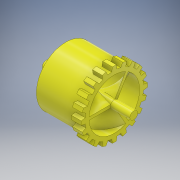
# Autodesk Inventor part: Rotator
Saved by Autodesk Inventor 2018.3 (Build 223284000, 284)
## iProperties
Created: 2020-03-27
Part Number: Rotator
Material: Generic
Document SubType Name: Modeling
Designer: ToreDenStore
Density: 1 g/cm^3
Appearance: Default
Author: ToreDenStore
Autodesk Inventor part; units mm, degrees
ref_plane "YZ Plane" through (0, 0, 0) normal (1, 0, 0) x (0, 1, 0)
ref_plane "XZ Plane" through (0, 0, 0) normal (0, 1, 0) x (-1, 0, 0)
ref_plane "XY Plane" through (0, 0, 0) normal (0, 0, 1) x (1, 0, 0)
sketch "Sketch1" plane through (0, 0, 0) normal (1, 0, 0) x (0, 1, 0)
  arc A0 (-7.1387, 10.8646) -> (-7.1387, -10.8646) centre (0, 0) ccw
  arc A1 (1.854, -0.75) -> (1.854, 0.75) centre (0, 0) ccw construction
  line L0 (12.9783, 0.75) -> (1.854, 0.75)
  line L1 (12.9783, -0.75) -> (1.854, -0.75)
  line L2 (-18.7818, 0) -> (21.6908, 0) projected
  line L3 (-7.1387, 10.8646) -> (-1.5765, 1.2307)
  line L4 (-5.8397, 11.6146) -> (-0.2775, 1.9807)
  line L5 (-5.8397, -11.6146) -> (-0.2775, -1.9807)
  line L6 (-7.1387, -10.8646) -> (-1.5765, -1.2307)
  arc A2 (-0.2775, -1.9807) -> (1.854, -0.75) centre (0, 0) ccw
  arc A3 (1.854, 0.75) -> (-0.2775, 1.9807) centre (0, 0) ccw
  arc A4 (-0.2775, 1.9807) -> (-1.5765, 1.2307) centre (0, 0) ccw construction
  arc A5 (-1.5765, 1.2307) -> (-1.5765, -1.2307) centre (0, 0) ccw
  arc A6 (-1.5765, -1.2307) -> (-0.2775, -1.9807) centre (0, 0) ccw construction
  arc A7 (-5.8397, 11.6146) -> (-7.1387, 10.8646) centre (0, 0) ccw
  arc A8 (-7.1387, -10.8646) -> (-5.8397, -11.6146) centre (0, 0) ccw
  arc A9 (-5.8397, -11.6146) -> (12.9783, -0.75) centre (0, 0) ccw
  arc A10 (12.9783, -0.75) -> (13, 0) centre (0, 0) ccw
  arc A11 (12.9783, 0.75) -> (-5.8397, 11.6146) centre (0, 0) ccw
  arc A12 (13, 0) -> (12.9783, 0.75) centre (0, 0) ccw
  dimension "d1" = 26
  dimension "d2" = 4
  dimension "d4" = 1.5
  dimension "d5" = 0.75
  dimension "d8" = 360
  constraints: 31 point on circle, 13 centre point, 12 end point, 2 parallel, 1 coincident, 1 point on line, 19 other
  measures "d1" diameter of A0
  measures "d2" diameter of A1
  measures "d4" distance between parallel lines of L0 L1
  measures "d5" distance between parallel lines of L2 L1
coil "Coil1" sketch "Sketch1" operation add axis through (-10, 0, 0) along (1, 0, 0) pitch 50 turns 0.5 hand right contours A7 L4 A3 L0 A12 L2 A5 L3 | L6 A5 L2 A10 L1 A2 L5 A8
sketch "Sketch2" plane through (25, -12.9783, -0.75) normal (1, 0, 0) x (0, 0, -1)
  circle A0 centre (-0.75, 12.9783) radius 15
  circle A1 centre (-0.75, 12.9783) radius 13
  dimension "d18" = 30
  dimension "d19" = 26
  constraints: 2 centre point, 2 coincident
  measures "d18" diameter of A0
  measures "d19" diameter of A1
extrude "Extrusion1" add sketch "Sketch2" against normal blind 25
sketch "Sketch3" plane through (25, 0, 0) normal (1, 0, 0) x (0, 0, -1)
  circle A0 centre (0, 0) radius 15 projected
  line L0 (0, 0) -> (-17, 0) construction
  line L1 (-17, 0) -> (-17, 1)
  line L2 (-17, 1) -> (-14.9379, 1.3636)
  line L3 (-17, 0) -> (-17, -1)
  line L4 (-17, -1) -> (-14.9379, -1.3636)
  circle A1 centre (0, 0) radius 15 construction
  line L5 (-14.9379, -1.3636) -> (-14.9379, 1.3636)
  dimension "d26" = 17
  dimension "d27" = 1
  dimension "d28" = 100
  constraints: 12 end point, 2 symmetric about line, 2 vertical, 1 horizontal, 2 other
  measures "d26" distance of L0.start L0.end
  measures "d27" distance of L0.end L1.end
  measures "d28" angle of L2 L1
extrude "Extrusion2" add sketch "Sketch3" against normal blind 5 contours L5 A0 | A0 L4 L3 L1 L2 picked at (-14.9563, 0.1517)
pattern_circular "Circular Pattern1" count 20 over 360 about axis through (-10, 0, 0) along (1, 0, 0) of "Extrusion2"
sketch "Sketch4" plane through (25, -1, 17) normal (1, 0, 0) x (0, 0, -1)
  circle A0 centre (17, 1) radius 2
  dimension "d34" = 4
  constraints: 1 centre point, 1 coincident
  measures "d34" diameter of A0
extrude "Extrusion3" add sketch "Sketch4" along normal blind 10
ref_plane "Mirror plane" through (12.5, -1, 17) normal (1, 0, 0) x (0, 0, -1)
mirror "Mirror1" about plane through (12.5, -1, 17) normal (1, 0, 0) of "Extrusion3"
equation "\"d5\" = 0.5 * d4"
body "Solid1"
